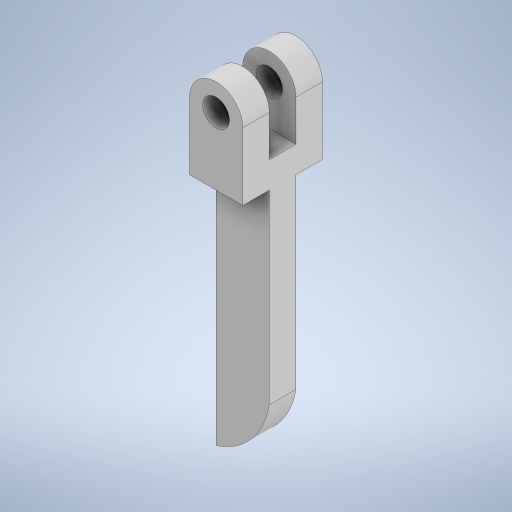
# Autodesk Inventor part: foot
Saved by Autodesk Inventor 2024 (Build 280153000, 153)
## iProperties
Created: 2024-08-23
Part Number: foot
Material: Generic
Document SubType Name: Modeling
Designer: domko
Density: 1 g/cm^3
Appearance: Default
Author: domko
Autodesk Inventor part; units mm, degrees
ref_plane "YZ Plane" through (0, 0, 0) normal (1, 0, 0) x (0, 1, 0)
ref_plane "XZ Plane" through (0, 0, 0) normal (0, 1, 0) x (-1, 0, 0)
ref_plane "XY Plane" through (0, 0, 0) normal (0, 0, 1) x (1, 0, 0)
sketch "Sketch1" plane through (0, 0, 0) normal (0, 0, 1) x (1, 0, 0)
  line L0 (-10, 43.5021) -> (10, 43.5021)
  line L1 (10, 43.5021) -> (10, -36.4979)
  line L2 (10, -36.4979) -> (-10, -36.4979)
  line L3 (-10, -36.4979) -> (-10, 43.5021)
  arc A0 (-10, -59.7738) -> (10, -36.4979) centre (-19.0329, -31.7817) ccw
  line L4 (-10, -59.7738) -> (-10, -36.4979)
  point P0 (0, 0)
  dimension "d0" = 20
  dimension "d1" = 10
  dimension "d2" = 80
  constraints: 10 end point, 2 parallel, 2 point on circle, 1 centre point, 1 collinear, 1 horizontal, 1 perpendicular
  measures "d0" distance between parallel lines of L1 L3
  measures "d1" distance from line of point (0, 0) L3
  measures "d2" distance of L0.end L1.end
extrude "Extrusion1" add sketch "Sketch1" along normal blind 10
sketch "Sketch2" plane through (0, 0, 10) normal (0, 0, 1) x (1, 0, 0)
  line L0 (-10, 43.5021) -> (-10, -59.7738) projected
  line L1 (-10, 33.5021) -> (10, 33.5021)
  line L2 (10, 33.5021) -> (10, 58.8152)
  line L3 (-10, 58.8152) -> (-10, 33.5021)
  line L4 (10, 43.5021) -> (-10, 43.5021) projected
  arc A0 (10, 58.8152) -> (-10, 58.8152) centre (0, 58.8152) ccw
  circle A1 centre (0, 58.8152) radius 5
  point P0 (0, 0)
  dimension "d5" = 20
  dimension "d6" = 10
  dimension "d7" = 10
  constraints: 6 end point, 2 centre point, 2 point on circle, 2 tangent, 1 coincident, 1 horizontal, 1 parallel, 1 perpendicular, 1 point on line
  measures "d5" distance of L1.start L1.end
  measures "d6" distance between parallel lines of L4 L1
  measures "d7" diameter of A1
extrude "Extrusion2" add sketch "Sketch2" along normal blind 10
sketch "Sketch3" plane through (0, 0, 0) normal (0, 0, -1) x (-1, 0, 0)
  point P0 (0, 0)
sketch "Sketch4" plane through (0, 0, 0) normal (0, 0, -1) x (-1, 0, 0)
  line L0 (-10, -36.4979) -> (-10, 43.5021) projected
  arc A0 (10, 58.8152) -> (-10, 58.8152) centre (0, 58.8152) ccw projected
  line L1 (-10, 33.5021) -> (10, 33.5021)
  line L2 (10, 33.5021) -> (10, 58.8152)
  line L3 (-10, 58.8152) -> (-10, 33.5021)
  line L4 (-10, 43.5021) -> (10, 43.5021) projected
  arc A1 (10, 58.8152) -> (-10, 58.8152) centre (0, 58.8152) ccw
  circle A2 centre (0, 58.8152) radius 5
  point P0 (0, 0)
  point P1 (-10, 58.8152)
  dimension "d10" = 10
  constraints: 6 end point, 3 point on circle, 2 centre point, 2 tangent, 1 coincident, 1 horizontal, 1 parallel, 1 perpendicular, 1 point on line
  measures "d10" distance between parallel lines of L4 L1
extrude "Extrusion3" add sketch "Sketch4" along normal blind 10
body "Solid1"
